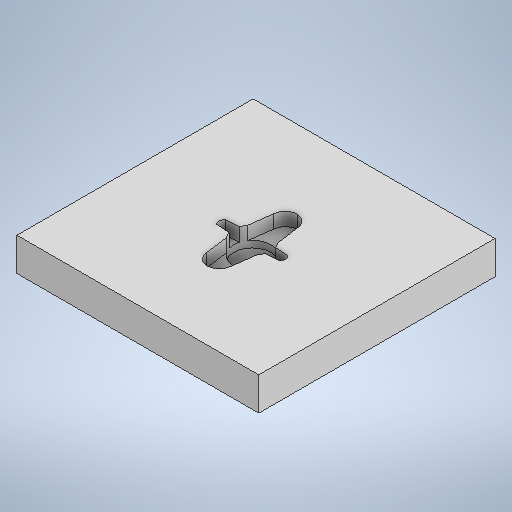
# Autodesk Inventor part: Part2
Saved by Autodesk Inventor 2025.1 (Build 291241000, 241)
## iProperties
Created: 2025-09-12
Part Number: Part2
Material: Generic
Document SubType Name: Modeling
Designer: nbro174
Density: 1 g/cm^3
Appearance: Default
Author: nbro174
Autodesk Inventor part; units mm, degrees
ref_plane "YZ Plane" through (0, 0, 0) normal (1, 0, 0) x (0, 1, 0)
ref_plane "XZ Plane" through (0, 0, 0) normal (0, 1, 0) x (-1, 0, 0)
ref_plane "XY Plane" through (0, 0, 0) normal (0, 0, 1) x (1, 0, 0)
sketch "Sketch1" plane through (0, 0, 0) normal (0, 1, 0) x (-1, 0, 0)
  line L0 (46.6892, 43.4449) -> (-45.937, 43.4449)
  line L1 (-45.937, 43.4449) -> (-45.937, -47.0251)
  line L2 (-45.937, -47.0251) -> (46.6892, -47.0251)
  line L3 (46.6892, -47.0251) -> (46.6892, 43.4449)
  point P0 (0, 0)
  constraints: 8 end point, 2 parallel, 1 horizontal, 1 perpendicular
extrude "Extrusion1" add sketch "Sketch1" along normal blind 12.7
sketch "Sketch2" plane through (0, 12.7, 0) normal (0, 1, 0) x (1, 0, 0)
  line L0 (-4.6344, -12.9521) -> (-6.35, -0.0003)
  line L1 (-4.6344, -12.9521) -> (0.0041, -12.9521)
  line L2 (0.0041, -12.9521) -> (4.5761, -12.9521)
  line L3 (4.5761, -12.9521) -> (6.35, -0.0003)
  arc A0 (0.004, -17.2664) -> (4.5761, -12.9521) centre (-0.3869, -12.2723) ccw
  arc A1 (-4.6344, -12.9521) -> (0.004, -17.2664) centre (0.1159, -12.4955) ccw
  line L4 (-4.6401, 12.8677) -> (0.0124, 12.8677)
  line L5 (0.0124, 12.8677) -> (4.5844, 12.8677)
  arc A2 (0.0041, 17.2458) -> (-4.6401, 12.8677) centre (0.1159, 12.4749) ccw
  arc A3 (4.5844, 12.8677) -> (0.0041, 17.2458) centre (-0.3881, 12.2505) ccw
  line L6 (4.5844, 12.8677) -> (6.35, -0.0003)
  line L7 (-4.6401, 12.8677) -> (-6.35, -0.0003)
  line L8 (-6.35, -0.0003) -> (-12.7, -0.0003)
  line L9 (6.35, -0.0003) -> (12.7, -0.0003)
  arc A4 (-12.7, -0.0003) -> (-12.0319, -1.6197) centre (-10.414, -0.0048) ccw
  line L10 (-6.35, -2.0323) -> (-12.0319, -1.6197)
  line L11 (-6.35, 2.0317) -> (-12.0319, 1.6102)
  arc A5 (-12.0319, 1.6102) -> (-12.7, -0.0092) centre (-10.414, -0.0048) ccw
  line L12 (-6.35, -2.0323) -> (-6.0808, -2.0323)
  line L13 (-6.35, 2.0317) -> (-6.08, 2.0317)
  line L14 (6.35, -0.0003) -> (12.7, -0.0003)
  arc A6 (12.7, -0.0003) -> (12.0319, 1.6191) centre (10.414, 0.0041) ccw
  line L15 (6.35, 2.0317) -> (12.0319, 1.6191)
  line L16 (6.35, -2.0323) -> (12.0319, -1.6108)
  arc A7 (12.0319, -1.6108) -> (12.7, 0.0085) centre (10.414, 0.0041) ccw
  line L17 (6.35, -2.0323) -> (6.0717, -2.0323)
  line L18 (6.35, 2.0317) -> (6.0712, 2.0317)
  point P0 (0, 0)
  point P1 (0.6686, -44.2967)
  point P2 (0.0037, 25.7566)
  point P3 (-0.0257, 7.5764)
  point P4 (0.0037, -0.0211)
  point P5 (12.0319, 1.6191)
  dimension "d12" = 4.572
  dimension "d16" = 4.572
  dimension "d20" = 2.032
  dimension "d21" = 2.032
  dimension "d22" = 2.286
  dimension "d25" = 2.032
  constraints: 38 end point, 18 point on circle, 8 centre point, 7 horizontal, 6 point on line, 2 concentric, 1 symmetric about line, 1 tangent
  measures "d12" distance of L1.end L2.end
  measures "d16" distance of L4.end L5.end
  measures "d20" distance of L0.end L11.start
  measures "d21" distance of L0.end L10.start
  measures "d22" radius of A4
  measures "d25" distance of L14.start L16.start
extrude "Extrusion2" cut sketch "Sketch2" against normal blind 5.08
sketch "Sketch3" plane through (0, 12.7, 0) normal (0, 1, 0) x (1, 0, 0)
  circle A0 centre (0, 0) radius 7.112
  dimension "d30" = 14.224
  constraints: 1 centre point, 1 coincident
  measures "d30" diameter of A0
extrude "Extrusion3" cut sketch "Sketch3" against normal blind 7.62
body "Solid1"
